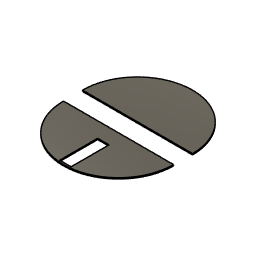
Lid Archive (Autodesk Fusion 360 design; units mm, degrees)
Autodesk Fusion 360 part; units mm, degrees
sketch "Lid" plane through (0, 0, 0) normal (0, 0, 1) x (1, 0, 0)
  arc A0 (145, 25.078) -> (-145, 24.922) centre (0, 25) ccw
  line L0 (0, 25) -> (145, 25.078) construction
  line L1 (0, 25) -> (-145, 24.922) construction
  arc A1 (-145, -25) -> (145, -25) centre (0, -25) ccw
  line L2 (0, -25) -> (-145, -25) construction
  line L3 (0, -25) -> (145, -25) construction
  line L4 (-15, -65) -> (15, -65)
  line L5 (15, -65) -> (15, -165)
  line L6 (15, -165) -> (-15, -165)
  line L7 (-15, -165) -> (-15, -65)
  line L8 (0, -25) -> (0, -65) construction
  line L9 (-145, -25) -> (145, -25)
  line L10 (-145, 24.922) -> (145, 25.078)
  dimension "d8" = 145
  dimension "d9" = 180
  dimension "d10" = 145
  dimension "d11" = 180
  dimension "d12" = 30
  dimension "d13" = 100
  dimension "d14" = 40
  constraint horizontal L4
  constraint vertical L5
  constraint horizontal L6
  constraint vertical L7
  constraint coincident A1.centre L2.start
  constraint perpendicular L4 L8
  measures "d8" radius of A0
  measures "d9" angle of L0 L1
  measures "d10" radius of A1
  measures "d11" angle of L2 L3
  measures "d12" distance of L4.start L4.end
  measures "d13" distance of L4.start L6.end
  measures "d14" distance of A1.centre L8.end
extrude "Extrude1" add sketch "Lid" along normal blind 3 makes body 1 at (34.8694, 65.0975, 0) makes body 2 at (-5, -38.3333, 0)
